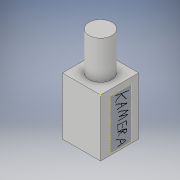
# Autodesk Inventor part: kamera_dummy
Saved by Autodesk Inventor 2017 (Build 210142000, 142)
## iProperties
Part Number: kamera_dummy
Material: Generisch
Document SubType Name: Modeling
Designer: Fabio
Density: 1 g/cm^3
Appearance: Vorgabe
Author: Fabio
Autodesk Inventor part; units mm, degrees
ref_plane "YZ Plane" through (0, 0, 0) normal (1, 0, 0) x (0, 1, 0)
ref_plane "XZ Plane" through (0, 0, 0) normal (0, 1, 0) x (-1, 0, 0)
ref_plane "XY Plane" through (0, 0, 0) normal (0, 0, 1) x (1, 0, 0)
sketch "Skizze1" plane through (0, 0, 0) normal (1, 0, 0) x (0, 1, 0)
  line L0 (0, 0) -> (20, 0)
  line L1 (20, 0) -> (20, -30)
  line L2 (20, -30) -> (0, -30)
  line L3 (0, -30) -> (0, 0)
  dimension "d0" = 20
  dimension "d1" = 30
  constraints: 8 end point, 2 parallel, 1 horizontal, 1 perpendicular
  measures "d0" distance of L1.end L2.end
  measures "d1" distance of L0.end L1.end
extrude "Extrusion1" add sketch "Skizze1" along normal blind 20
sketch "Skizze2" plane through (0, 0, 0) normal (0, 0, 1) x (1, 0, 0)
  line L0 (0, 20) -> (20, 20) construction
  line L1 (0, 0) -> (20, 20) construction
  line L2 (0, 20) -> (20, 0) construction
  line L3 (20, 20) -> (20, 0) construction
  circle A0 centre (10, 10) radius 6
  dimension "d4" = 12
  constraints: 5 end point, 1 centre point, 1 midpoint
  measures "d4" diameter of A0
extrude "Extrusion2" add sketch "Skizze2" along normal blind 20
sketch "Skizze3" plane through (20, 0, 0) normal (1, 0, 0) x (0, 0, -1)
  line L0 (3.2137, 16.0634) -> (29.2155, 16.0634) construction
  line L1 (29.2155, 16.0634) -> (29.2155, 5.0626) construction
  line L2 (29.2155, 5.0626) -> (3.2137, 5.0626) construction
  line L3 (3.2137, 5.0626) -> (3.2137, 16.0634) construction
  point P0 (0, 0)
  constraints: 2 other
